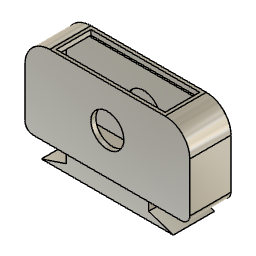
slider v1 (Autodesk Fusion 360 design; units mm, degrees)
Autodesk Fusion 360 part; units mm, degrees
note: some values were not read from the file. Set by a fixed rule: which sketch regions a step uses.
sketch "Sketch1" plane through (0, 0, 0) normal (0, 1, 0) x (1, 0, 0)
  line L0 (0, -35) -> (0, 22.8292) construction
  line L1 (25, 0) -> (25, 5)
  line L2 (25, 5) -> (40, 10)
  line L3 (40, 10) -> (0, 10)
  line L4 (-25, 0) -> (-25, 5)
  line L5 (-25, 5) -> (-40, 10)
  line L6 (-40, 10) -> (0, 10)
  line L7 (25, 0) -> (45, 0)
  line L8 (50, -5) -> (50, -35)
  line L9 (35, -50) -> (-35, -50)
  line L10 (-50, -35) -> (-50, -5)
  line L11 (-45, 0) -> (-25, 0)
  circle A0 centre (0, -25) radius 10
  arc A1 (35, -50) -> (50, -35) centre (35, -35) ccw
  arc A2 (-50, -35) -> (-35, -50) centre (-35, -35) ccw
  arc A3 (-45, 0) -> (-50, -5) centre (-45, -5) ccw
  arc A4 (50, -5) -> (45, 0) centre (45, -5) ccw
  point P0 (50, 0)
  point P1 (50, -50)
  dimension "d5" = 40
  dimension "d6" = 5
  dimension "d7" = 25
  dimension "d8" = 5
  dimension "d9" = 50
  dimension "d10" = 20
  dimension "d11" = 25
  dimension "d14" = 15
  dimension "d15" = 15
  dimension "d16" = 5
  dimension "d17" = 5
  constraint vertical L0
  constraint coincident L0 L3.end
  constraint perpendicular L0 L3
  constraint coincident origin L0
  constraint symmetric L0 L1.start L4.start
  constraint symmetric L0 L1.end L4.end
  constraint symmetric L0 L2.end L5.end
  constraint symmetric L0 L3.end L6.end
  constraint perpendicular L1 L7
  constraint perpendicular L7 L8
  constraint perpendicular L8 L9
  constraint perpendicular L9 L10
  constraint perpendicular L4 L11
  constraint coincident L0 A0.centre
  constraint coincident P1 L8
  constraint coincident P1 L9
  constraint tangent L8 A1
  constraint tangent L9 A1
  constraint tangent L9 A2
  constraint tangent L10 A2
  constraint tangent L10 A3
  constraint tangent L11 A3
  constraint coincident P0 L8
  constraint coincident P0 L7
  constraint tangent L8 A4
  constraint tangent L7 A4
  measures "d5" distance of L2.end L3.end
  measures "d6" distance of L1.start L1.end
  measures "d7" distance of origin L1.start
  measures "d8" distance of L1.end L3
  measures "d9" distance of P0 P1
  measures "d10" diameter of A0
  measures "d11" distance of L9 A0.centre
  measures "d14" radius of A1
  measures "d15" radius of A2
  measures "d16" radius of A3
  measures "d17" radius of A4
extrude "Extrude1" add sketch "Sketch1" along normal blind 25 contours L1 L2 L3 L4 L5 L6 L7 L8 L9 L10 L11 A1 A2 A3 A4 | A0 makes body 1
split "Split1" by plane through (25, 0, 0) normal (0, 0, -1) bodies 1 makes body 2 at (26.6667, 8.3333, -10)
sketch "Sketch2" plane through (0, 0, 50) normal (0, 0, 1) x (-1, 0, 0)
  line L0 (35, 0) -> (-35, 0)
  line L1 (-35, 0) -> (-35, -25)
  line L2 (-35, -25) -> (35, -25)
  line L3 (35, -25) -> (35, 0)
  line L4 (33, -2) -> (-33, -2)
  line L5 (-33, -2) -> (-33, -23)
  line L6 (-33, -23) -> (33, -23)
  line L7 (33, -23) -> (33, -2)
  dimension "d18" = -2
extrude "Extrude2" cut sketch "Sketch2" against normal blind 3 contours L4 L5 L6 L7 bodies 1
shell "Shell1" thickness 3 removed faces 1 at (11, 9, 47) on bodies 1
extrude "Extrude3" cut sketch "Sketch1" along normal blind 23 contours A0 bodies 1
